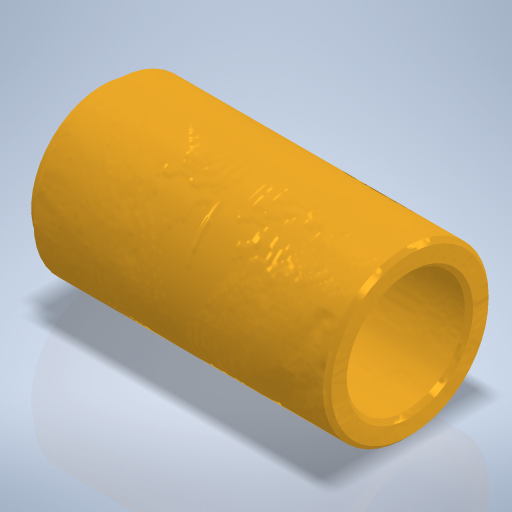
# Autodesk Inventor part: Ak zylinder
Saved by Autodesk Inventor 2024 (Build 280153000, 153)
## iProperties
Created: 2024-04-02
Part Number: Ak zylinder
Material: Messing, weicher Gelbton, geschweißt
Document SubType Name: Modeling
Designer: ffogue
Density: 8.5 g/cm^3
Appearance: Schweißnaht - Messing
Author: ffogue
Autodesk Inventor part; units mm, degrees
ref_plane "YZ Plane" through (0, 0, 0) normal (1, 0, 0) x (0, 1, 0)
ref_plane "XZ Plane" through (0, 0, 0) normal (0, 1, 0) x (-1, 0, 0)
ref_plane "XY Plane" through (0, 0, 0) normal (0, 0, 1) x (1, 0, 0)
sketch "Skizze2" plane through (0, 0, 0) normal (0, 0, 1) x (1, 0, 0)
  line L0 (0, 0) -> (0, 6)
  line L1 (0, 6) -> (1.2, 6)
  line L2 (1.2, 6) -> (1.2, 7)
  line L3 (1.2, 7) -> (26, 7)
  line L4 (26, 7) -> (26, 0)
  line L5 (26, 0) -> (0, 0)
  dimension "d0" = 26
  dimension "d1" = 14
  dimension "d2" = 12
  dimension "d3" = 1.2
  constraints: 12 end point, 5 perpendicular, 1 vertical
  measures "d0" distance of L4.end L0.start
  measures "d1" diameter of L3 L5
  measures "d2" diameter of L1 L5
  measures "d3" distance from line of L2.end L0
revolve "Umdrehung1" add sketch "Skizze2" angle 360 about axis through (26, 0, 0) along (-1, 0, 0)
sketch "Skizze3" plane through (0, 0, 0) normal (-1, 0, 0) x (0, 0, 1)
  circle A0 centre (0, 0) radius 5
  dimension "d5" = 10
  constraints: 1 centre point, 1 coincident
  measures "d5" diameter of A0
extrude "Extrusion1" cut sketch "Skizze3" against normal up to surface (26 mm away)
chamfer "Fasen1" distance 0.35 angle 45 2 edges at (26, 0, -5) (26, -7, 0)
